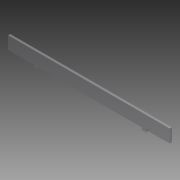
# Autodesk Inventor part: Funneling 4
Saved by Autodesk Inventor 2013 (Build 170138000, 138)
## iProperties
Created: 2013-01-26
Part Number: Funneling 4
Material: Polycarbonate, Clear
Document SubType Name: Modeling
Designer: actoennies
Mass: 103.924 g
Surface Area: 433.064 cm^2
Volume: 116.246 cm^3
Density: 0.894 g/cm^3
Author: actoennies
Autodesk Inventor part; units mm, degrees
ref_plane "YZ Plane" through (0, 0, 0) normal (1, 0, 0) x (0, 1, 0)
ref_plane "XZ Plane" through (0, 0, 0) normal (0, 1, 0) x (-1, 0, 0)
ref_plane "XY Plane" through (0, 0, 0) normal (0, 0, 1) x (1, 0, 0)
sketch "Sketch1" plane through (0, 0, 0) normal (0, 0, 1) x (1, 0, 0)
  line L0 (0, 0) -> (0, 38.1)
  line L1 (0, 0) -> (76.2, 0)
  line L2 (76.2, 0) -> (76.2, -6.35)
  line L3 (76.2, -6.35) -> (88.9, -6.35)
  line L4 (88.9, -6.35) -> (88.9, 0)
  line L5 (88.9, 0) -> (393.7, 0)
  line L6 (393.7, 0) -> (393.7, -6.35)
  line L7 (393.7, -6.35) -> (406.4, -6.35)
  line L8 (406.4, -6.35) -> (406.4, 0)
  line L9 (0, 38.1) -> (476.25, 38.1)
  line L10 (406.4, 0) -> (476.25, 0)
  line L11 (476.25, 0) -> (476.25, 38.1)
  dimension "d0" = 38.1
  dimension "d1" = 76.2
  dimension "d2" = 6.35
  dimension "d3" = 12.7
  dimension "d4" = 304.8
  dimension "d5" = 12.7
  dimension "d6" = 476.25
  constraints: 24 end point, 7 perpendicular, 3 parallel, 2 point on line, 1 vertical
  measures "d0" distance of L0.start L0.end
  measures "d1" distance of L0.start L1.end
  measures "d2" distance of L1.end L2.end
  measures "d3" distance of L2.end L3.end
  measures "d4" distance of L4.end L5.end
  measures "d5" distance of L6.end L7.end
  measures "d6" distance of L0.end L9.end
extrude "Extrusion1" add sketch "Sketch1" along normal blind 6.35
body "Solid1"
